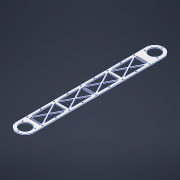
# Autodesk Inventor part: Lower_Arm_Bearing_Side
Saved by Autodesk Inventor 2022 (Build 260153000, 153)
## iProperties
Created: 2023-02-15
Part Number: Lower_Arm_Bearing_Side
Material: Aluminum 6061
Document SubType Name: Modeling
Designer: dzw04
Density: 2.7 g/cm^3
Appearance: Aluminum - Flat
Author: dzw04
Autodesk Inventor part; units mm, degrees
ref_plane "YZ Plane" through (0, 0, 0) normal (1, 0, 0) x (0, 1, 0)
ref_plane "XZ Plane" through (0, 0, 0) normal (0, 1, 0) x (-1, 0, 0)
ref_plane "XY Plane" through (0, 0, 0) normal (0, 0, 1) x (1, 0, 0)
sketch "Sketch1" plane through (0, 0, 0) normal (0, 1, 0) x (-1, 0, 0)
  line L0 (27.5, 400) -> (27.5, 0)
  arc A0 (-27.5, 0) -> (27.5, 0) centre (0, 0) ccw
  line L1 (-27.5, 0) -> (-27.5, 400)
  arc A1 (27.5, 400) -> (-27.5, 400) centre (0, 400) ccw
  circle A2 centre (23.5, 370) radius 1.5
  circle A3 centre (-23.25, 370) radius 1.5
  circle A4 centre (0, 422) radius 1.5
  circle A5 centre (0, 400) radius 17.5
  circle A6 centre (-19.0526, 389) radius 1.5
  circle A7 centre (19.0526, 389) radius 1.5
  arc A8 (16.4763, 364.5362) -> (15.5903, 366) centre (15.5903, 365) ccw
  line L2 (15.5903, 366) -> (-15.5903, 366)
  arc A9 (-15.5903, 366) -> (-16.4763, 364.5362) centre (-15.5903, 365) ccw
  line L3 (-16.4763, 364.5362) -> (-0.8859, 334.7547)
  arc A10 (-0.8859, 334.7547) -> (0.8859, 334.7547) centre (0, 335.2185) ccw
  line L4 (0.8859, 334.7547) -> (16.4763, 364.5362)
  circle A11 centre (-23.25, 328.75) radius 1.5
  arc A12 (16.4763, 282.0362) -> (15.5903, 283.5) centre (15.5903, 282.5) ccw
  line L5 (15.5903, 283.5) -> (-15.5903, 283.5)
  arc A13 (-15.5903, 283.5) -> (-16.4763, 282.0362) centre (-15.5903, 282.5) ccw
  line L6 (-16.4763, 282.0362) -> (-0.8859, 252.2547)
  arc A14 (-0.8859, 252.2547) -> (0.8859, 252.2547) centre (0, 252.7185) ccw
  line L7 (0.8859, 252.2547) -> (16.4763, 282.0362)
  circle A15 centre (-23.25, 205) radius 1.5
  circle A16 centre (-23.25, 287.5) radius 1.5
  circle A17 centre (-23.25, 246.25) radius 1.5
  line L8 (15.5903, 118.5) -> (-15.5903, 118.5)
  arc A18 (-15.5903, 118.5) -> (-16.4763, 117.0362) centre (-15.5903, 117.5) ccw
  line L9 (-16.4763, 117.0362) -> (-0.8859, 87.2547)
  arc A19 (-0.8859, 87.2547) -> (0.8859, 87.2547) centre (0, 87.7185) ccw
  line L10 (0.8859, 87.2547) -> (16.4763, 117.0362)
  arc A20 (16.4763, 117.0362) -> (15.5903, 118.5) centre (15.5903, 117.5) ccw
  circle A21 centre (-23.25, 122.5) radius 1.5
  circle A22 centre (-23.25, 81.25) radius 1.5
  arc A23 (-2.5003, 328.2862) -> (-2.5003, 329.2138) centre (-3.3862, 328.75) ccw
  line L11 (-2.5003, 329.2138) -> (-17.6141, 358.085)
  arc A24 (-17.6141, 358.085) -> (-19.5, 357.6212) centre (-18.5, 357.6212) ccw
  line L12 (-19.5, 357.6212) -> (-19.5, 299.8788)
  arc A25 (-19.5, 299.8788) -> (-17.6141, 299.415) centre (-18.5, 299.8788) ccw
  line L13 (-17.6141, 299.415) -> (-2.5003, 328.2862)
  line L14 (16.4763, 45.4638) -> (0.8859, 75.2453)
  arc A26 (0.8859, 75.2453) -> (-0.8859, 75.2453) centre (0, 74.7815) ccw
  line L15 (-0.8859, 75.2453) -> (-16.4763, 45.4638)
  arc A27 (-16.4763, 45.4638) -> (-15.5903, 44) centre (-15.5903, 45) ccw
  line L16 (-15.5903, 44) -> (15.5903, 44)
  arc A28 (15.5903, 44) -> (16.4763, 45.4638) centre (15.5903, 45) ccw
  arc A29 (17.6141, 299.415) -> (19.5, 299.8788) centre (18.5, 299.8788) ccw
  line L17 (19.5, 299.8788) -> (19.5, 357.6212)
  arc A30 (19.5, 357.6212) -> (17.6141, 358.085) centre (18.5, 357.6212) ccw
  line L18 (17.6141, 358.085) -> (2.5003, 329.2138)
  arc A31 (2.5003, 329.2138) -> (2.5003, 328.2862) centre (3.3862, 328.75) ccw
  line L19 (2.5003, 328.2862) -> (17.6141, 299.415)
  line L20 (2.5003, 245.7862) -> (17.6141, 216.915)
  arc A32 (17.6141, 216.915) -> (19.5, 217.3788) centre (18.5, 217.3788) ccw
  line L21 (19.5, 217.3788) -> (19.5, 275.1212)
  arc A33 (19.5, 275.1212) -> (17.6141, 275.585) centre (18.5, 275.1212) ccw
  line L22 (17.6141, 275.585) -> (2.5003, 246.7138)
  arc A34 (2.5003, 246.7138) -> (2.5003, 245.7862) centre (3.3862, 246.25) ccw
  arc A35 (15.5903, 291.5) -> (16.4763, 292.9638) centre (15.5903, 292.5) ccw
  line L23 (16.4763, 292.9638) -> (0.8859, 322.7453)
  arc A36 (0.8859, 322.7453) -> (-0.8859, 322.7453) centre (0, 322.2815) ccw
  line L24 (-0.8859, 322.7453) -> (-16.4763, 292.9638)
  arc A37 (-16.4763, 292.9638) -> (-15.5903, 291.5) centre (-15.5903, 292.5) ccw
  line L25 (-15.5903, 291.5) -> (15.5903, 291.5)
  circle A38 centre (23.5, 246.25) radius 1.5
  line L26 (-17.6141, 51.915) -> (-2.5003, 80.7862)
  arc A39 (-2.5003, 80.7862) -> (-2.5003, 81.7138) centre (-3.3862, 81.25) ccw
  line L27 (-2.5003, 81.7138) -> (-17.6141, 110.585)
  arc A40 (-17.6141, 110.585) -> (-19.5, 110.1212) centre (-18.5, 110.1212) ccw
  line L28 (-19.5, 110.1212) -> (-19.5, 52.3788)
  arc A41 (-19.5, 52.3788) -> (-17.6141, 51.915) centre (-18.5, 52.3788) ccw
  arc A42 (-15, 206.5) -> (-15, 203.5) centre (-15, 205) ccw
  line L29 (-15, 203.5) -> (15, 203.5)
  arc A43 (15, 203.5) -> (15, 206.5) centre (15, 205) ccw
  line L30 (15, 206.5) -> (-15, 206.5)
  line L31 (2.5003, 80.7862) -> (17.6141, 51.915)
  arc A44 (17.6141, 51.915) -> (19.5, 52.3788) centre (18.5, 52.3788) ccw
  line L32 (19.5, 52.3788) -> (19.5, 110.1212)
  arc A45 (19.5, 110.1212) -> (17.6141, 110.585) centre (18.5, 110.1212) ccw
  line L33 (17.6141, 110.585) -> (2.5003, 81.7138)
  arc A46 (2.5003, 81.7138) -> (2.5003, 80.7862) centre (3.3862, 81.25) ccw
  line L34 (0.8859, 169.7547) -> (16.4763, 199.5362)
  arc A47 (16.4763, 199.5362) -> (15.5903, 201) centre (15.5903, 200) ccw
  line L35 (15.5903, 201) -> (-15.5903, 201)
  arc A48 (-15.5903, 201) -> (-16.4763, 199.5362) centre (-15.5903, 200) ccw
  line L36 (-16.4763, 199.5362) -> (-0.8859, 169.7547)
  arc A49 (-0.8859, 169.7547) -> (0.8859, 169.7547) centre (0, 170.2185) ccw
  circle A50 centre (23.5, 81.25) radius 1.5
  circle A51 centre (23.5, 328.75) radius 1.5
  line L37 (-0.8859, 157.7453) -> (-16.4763, 127.9638)
  arc A52 (-16.4763, 127.9638) -> (-15.5903, 126.5) centre (-15.5903, 127.5) ccw
  line L38 (-15.5903, 126.5) -> (15.5903, 126.5)
  arc A53 (15.5903, 126.5) -> (16.4763, 127.9638) centre (15.5903, 127.5) ccw
  line L39 (16.4763, 127.9638) -> (0.8859, 157.7453)
  arc A54 (0.8859, 157.7453) -> (-0.8859, 157.7453) centre (0, 157.2815) ccw
  arc A55 (-17.6141, 275.585) -> (-19.5, 275.1212) centre (-18.5, 275.1212) ccw
  line L40 (-19.5, 275.1212) -> (-19.5, 217.3788)
  arc A56 (-19.5, 217.3788) -> (-17.6141, 216.915) centre (-18.5, 217.3788) ccw
  line L41 (-17.6141, 216.915) -> (-2.5003, 245.7862)
  arc A57 (-2.5003, 245.7862) -> (-2.5003, 246.7138) centre (-3.3862, 246.25) ccw
  line L42 (-2.5003, 246.7138) -> (-17.6141, 275.585)
  arc A58 (0.8859, 240.2453) -> (-0.8859, 240.2453) centre (0, 239.7815) ccw
  line L43 (-0.8859, 240.2453) -> (-16.4763, 210.4638)
  arc A59 (-16.4763, 210.4638) -> (-15.5903, 209) centre (-15.5903, 210) ccw
  line L44 (-15.5903, 209) -> (15.5903, 209)
  arc A60 (15.5903, 209) -> (16.4763, 210.4638) centre (15.5903, 210) ccw
  line L45 (16.4763, 210.4638) -> (0.8859, 240.2453)
  circle A61 centre (23.5, 122.5) radius 1.5
  circle A62 centre (23.5, 205) radius 1.5
  line L46 (17.6141, 193.085) -> (2.5003, 164.2138)
  arc A63 (2.5003, 164.2138) -> (2.5003, 163.2862) centre (3.3862, 163.75) ccw
  line L47 (2.5003, 163.2862) -> (17.6141, 134.415)
  arc A64 (17.6141, 134.415) -> (19.5, 134.8788) centre (18.5, 134.8788) ccw
  line L48 (19.5, 134.8788) -> (19.5, 192.6212)
  arc A65 (19.5, 192.6212) -> (17.6141, 193.085) centre (18.5, 192.6212) ccw
  line L49 (-17.6141, 134.415) -> (-2.5003, 163.2862)
  arc A66 (-2.5003, 163.2862) -> (-2.5003, 164.2138) centre (-3.3862, 163.75) ccw
  line L50 (-2.5003, 164.2138) -> (-17.6141, 193.085)
  arc A67 (-17.6141, 193.085) -> (-19.5, 192.6212) centre (-18.5, 192.6212) ccw
  line L51 (-19.5, 192.6212) -> (-19.5, 134.8788)
  arc A68 (-19.5, 134.8788) -> (-17.6141, 134.415) centre (-18.5, 134.8788) ccw
  circle A69 centre (23.5, 287.5) radius 1.5
  circle A70 centre (-23.25, 163.75) radius 1.5
  circle A71 centre (23.5, 163.75) radius 1.5
  circle A72 centre (23.5, 40) radius 1.5
  line L52 (-15, 38.5) -> (15, 38.5)
  arc A73 (15, 38.5) -> (15, 41.5) centre (15, 40) ccw
  line L53 (15, 41.5) -> (-15, 41.5)
  arc A74 (-15, 41.5) -> (-15, 38.5) centre (-15, 40) ccw
  circle A75 centre (-23.25, 40) radius 1.5
  line L54 (15, 371.5) -> (-15, 371.5)
  arc A76 (-15, 371.5) -> (-15, 368.5) centre (-15, 370) ccw
  line L55 (-15, 368.5) -> (15, 368.5)
  arc A77 (15, 368.5) -> (15, 371.5) centre (15, 370) ccw
  circle A78 centre (0, -22) radius 1.5
  circle A79 centre (19.0526, 11) radius 1.5
  circle A80 centre (-19.0526, 11) radius 1.5
  circle A81 centre (0, 0) radius 17.5
  point P0 (15, 368.5)
  point P1 (-15, 368.5)
  point P2 (-15, 41.5)
  point P3 (-2.5003, 164.2138)
  point P4 (2.5003, 163.2862)
  point P5 (0.8859, 240.2453)
  point P6 (15.5903, 209)
  point P7 (-15.5903, 209)
  point P8 (-0.8859, 240.2453)
  point P9 (-17.6141, 275.585)
  point P10 (-2.5003, 246.7138)
  point P11 (-2.5003, 245.7862)
  point P12 (0.8859, 157.7453)
  point P13 (16.4763, 127.9638)
  point P14 (-16.4763, 199.5362)
  point P15 (19.5, 52.3788)
  point P16 (15, 206.5)
  point P17 (15, 203.5)
  point P18 (-2.5003, 81.7138)
  point P19 (-2.5003, 80.7862)
  point P20 (0.8859, 322.7453)
  point P21 (16.4763, 292.9638)
  point P22 (2.5003, 246.7138)
  point P23 (17.6141, 275.585)
  point P24 (19.5, 217.3788)
  point P25 (17.6141, 299.415)
  point P26 (2.5003, 328.2862)
  point P27 (17.6141, 358.085)
  point P28 (-0.8859, 75.2453)
  point P29 (-19.5, 357.6212)
  point P30 (0.8859, 87.2547)
  point P31 (-0.8859, 87.2547)
  point P32 (-15.5903, 118.5)
  point P33 (0.8859, 252.2547)
  point P34 (-16.4763, 282.0362)
  point P35 (-15.5903, 283.5)
  point P36 (16.4763, 364.5362)
  point P37 (0.8859, 334.7547)
  point P38 (-16.4763, 364.5362)
  constraints: 112 end point, 112 point on circle, 82 centre point
extrude "Extrusion1" add sketch "Sketch1" along normal blind 3
body "Solid1"
